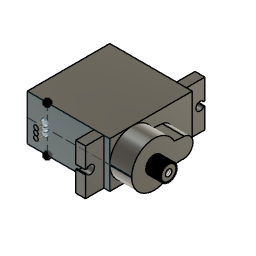
Arm_1 v1 (Autodesk Fusion 360 archive; units mm, degrees)
design "ServoMF90"
Autodesk Fusion 360 part; units mm, degrees
sketch "Sketch1" plane through (0, 0, 0) normal (0, 0, 1) x (1, 0, 0)
  line L0 (-11.3, 11.3) -> (11.3, 11.3)
  line L1 (11.3, 11.3) -> (11.3, -11.3)
  line L2 (11.3, -11.3) -> (-11.3, -11.3)
  line L3 (-11.3, -11.3) -> (-11.3, 11.3)
  line L4 (-11.3, 11.3) -> (11.3, -11.3) construction
  line L5 (11.3, 11.3) -> (-11.3, -11.3) construction
  dimension "d1" = 22.6
  dimension "d2" = 22.6
  constraint horizontal L0
  constraint perpendicular L0 L1
  constraint parallel L0 L2
  constraint parallel L1 L3
  constraint coincident L4 origin
  constraint coincident L5 origin
  measures "d1" distance of L1.end L2.end
  measures "d2" distance of L0.end L1.end
extrude "Extrude1" add sketch "Sketch1" along normal blind 12.5 contours L0 L1 L2 L3 picked at (-3.766667, 3.766667) makes body 1
sketch "Sketch2" plane through (11.3, 0, 0) normal (1, 0, 0) x (0, 1, 0)
  line L0 (-11.3, 0) -> (11.3, 0)
  line L1 (11.3, 0) -> (11.3, 12.5)
  line L2 (11.3, 12.5) -> (-11.3, 12.5)
  line L3 (-11.3, 12.5) -> (-11.3, 0)
  circle A0 centre (-5.148532, 6.347755) radius 6.152245
  line L4 (-5.148532, 6.347755) -> (11.3, 6.25) construction
  circle A1 centre (2.851468, 6.25) radius 2.65
  line L5 (3.075734, 8.890493) -> (0.342379, 9.122646)
  line L6 (3.075734, -8.890493) -> (0.342379, -9.122646)
  line L7 (3.044931, 3.707445) -> (0.309009, 3.507796)
  circle A2 centre (-5.148532, 6.347755) radius 2.3
  dimension "d5" = 5.3
  dimension "d6" = 8
  dimension "d7" = 4.6
  constraint tangent L2 A0
  constraint midpoint L1 L4.end
  constraint tangent A1 L5
  constraint concentric A0 A2
  measures "d5" diameter of A1
  measures "d7" diameter of A2
extrude "Extrude2" add sketch "Sketch2" along normal blind 6 contours A0 A1 | A0 A1 L7 | A0 A1 L5 | A0 A1 | A0 A1 picked at (-0.779294, 7.905006) picked at (0.801754, 3.761707) picked at (0.843844, 8.497494) picked at (0.728856, 6.066378) picked at (2.263353, 5.526518) bodies 1
extrude "Extrude3" add 1 faces at (11.3, -6.264471, 5.742797) along direction (1, 0, 0) blind 10 on bodies 1 bodies 1
sketch "Sketch3" plane through (21.3, 0, 0) normal (1, 0, 0) x (0, 1, 0)
  circle A0 centre (-5.148532, 6.347755) radius 2.3
  circle A1 centre (-5.148532, 6.347755) radius 1.1
  dimension "d12" = 2.2
  constraint concentric A0 A1
  measures "d12" diameter of A1
extrude "Extrude4" cut sketch "Sketch3" against normal blind 4 contours A1 picked at (-5.895648, 6.553327) bodies 1
thread "Thread1" "ISO Metric profile 2.2 M2.2x0.45 6H" major diameter 2.28 minor diameter 1.7754 pitch 0.45 angle 60 resizes the face on face at (19.966667, -4.053998, 6.23823) on bodies 1
sketch "Sketch4" plane through (21.3, 0, 0) normal (1, 0, 0) x (0, 1, 0)
  circle A0 centre (-5.148532, 6.347755) radius 0.8877
  circle A1 centre (-5.148532, 6.347755) radius 2.3
  line L0 (-5.287623, 4.051965) -> (-4.937623, 4.051965)
  line L1 (-4.937623, 4.051965) -> (-4.937623, 4.351965)
  line L2 (-4.937623, 4.351965) -> (-5.287623, 4.351965)
  line L3 (-5.287623, 4.351965) -> (-5.287623, 4.051965)
  line L4 (-4.766335, 4.38397) -> (-4.68869, 4.094192)
  line L5 (-4.428261, 4.474556) -> (-4.766335, 4.38397)
  line L6 (-4.350616, 4.184779) -> (-4.428261, 4.474556)
  line L7 (-4.68869, 4.094192) -> (-4.350616, 4.184779)
  line L8 (-4.271093, 4.549804) -> (-4.121093, 4.289996)
  line L9 (-3.967985, 4.724804) -> (-4.271093, 4.549804)
  line L10 (-3.817985, 4.464996) -> (-3.967985, 4.724804)
  line L11 (-4.121093, 4.289996) -> (-3.817985, 4.464996)
  line L12 (-3.835647, 4.838165) -> (-3.623515, 4.626033)
  line L13 (-3.58816, 5.085653) -> (-3.835647, 4.838165)
  line L14 (-3.376028, 4.873521) -> (-3.58816, 5.085653)
  line L15 (-3.623515, 4.626033) -> (-3.376028, 4.873521)
  line L16 (-3.489672, 5.229403) -> (-3.229865, 5.079403)
  line L17 (-3.314672, 5.532511) -> (-3.489672, 5.229403)
  line L18 (-3.054865, 5.382511) -> (-3.314672, 5.532511)
  line L19 (-3.229865, 5.079403) -> (-3.054865, 5.382511)
  line L20 (-3.256746, 5.696854) -> (-2.966968, 5.619208)
  line L21 (-3.166159, 6.034928) -> (-3.256746, 5.696854)
  line L22 (-2.876381, 5.957282) -> (-3.166159, 6.034928)
  line L23 (-2.966968, 5.619208) -> (-2.876381, 5.957282)
  line L24 (-3.152741, 6.208663) -> (-2.852741, 6.208663)
  line L25 (-3.152741, 6.558663) -> (-3.152741, 6.208663)
  line L26 (-2.852741, 6.558663) -> (-3.152741, 6.558663)
  line L27 (-2.852741, 6.208663) -> (-2.852741, 6.558663)
  line L28 (-3.184746, 6.729951) -> (-2.894969, 6.807597)
  line L29 (-3.275333, 7.068025) -> (-3.184746, 6.729951)
  line L30 (-2.985555, 7.145671) -> (-3.275333, 7.068025)
  line L31 (-2.894969, 6.807597) -> (-2.985555, 7.145671)
  line L32 (-3.35058, 7.225193) -> (-3.090773, 7.375193)
  line L33 (-3.52558, 7.528302) -> (-3.35058, 7.225193)
  line L34 (-3.265773, 7.678302) -> (-3.52558, 7.528302)
  line L35 (-3.090773, 7.375193) -> (-3.265773, 7.678302)
  line L36 (-3.638942, 7.660639) -> (-3.42681, 7.872771)
  line L37 (-3.886429, 7.908126) -> (-3.638942, 7.660639)
  line L38 (-3.674297, 8.120258) -> (-3.886429, 7.908126)
  line L39 (-3.42681, 7.872771) -> (-3.674297, 8.120258)
  line L40 (-4.030179, 8.006614) -> (-3.880179, 8.266422)
  line L41 (-4.333288, 8.181614) -> (-4.030179, 8.006614)
  line L42 (-4.183288, 8.441422) -> (-4.333288, 8.181614)
  line L43 (-3.880179, 8.266422) -> (-4.183288, 8.441422)
  line L44 (-4.497631, 8.239541) -> (-4.419985, 8.529318)
  line L45 (-4.835705, 8.330127) -> (-4.497631, 8.239541)
  line L46 (-4.758059, 8.619905) -> (-4.835705, 8.330127)
  line L47 (-4.419985, 8.529318) -> (-4.758059, 8.619905)
  line L48 (-5.00944, 8.343545) -> (-5.00944, 8.643545)
  line L49 (-5.35944, 8.343545) -> (-5.00944, 8.343545)
  line L50 (-5.35944, 8.643545) -> (-5.35944, 8.343545)
  line L51 (-5.00944, 8.643545) -> (-5.35944, 8.643545)
  line L52 (-5.530728, 8.31154) -> (-5.608373, 8.601318)
  line L53 (-5.868802, 8.220953) -> (-5.530728, 8.31154)
  line L54 (-5.946447, 8.510731) -> (-5.868802, 8.220953)
  line L55 (-5.608373, 8.601318) -> (-5.946447, 8.510731)
  line L56 (-6.02597, 8.145706) -> (-6.17597, 8.405514)
  line L57 (-6.329079, 7.970706) -> (-6.02597, 8.145706)
  line L58 (-6.479079, 8.230514) -> (-6.329079, 7.970706)
  line L59 (-6.17597, 8.405514) -> (-6.479079, 8.230514)
  line L60 (-6.461416, 7.857345) -> (-6.673548, 8.069477)
  line L61 (-6.708903, 7.609857) -> (-6.461416, 7.857345)
  line L62 (-6.921035, 7.821989) -> (-6.708903, 7.609857)
  line L63 (-6.673548, 8.069477) -> (-6.921035, 7.821989)
  line L64 (-6.807391, 7.466107) -> (-7.067198, 7.616107)
  line L65 (-6.982391, 7.162998) -> (-6.807391, 7.466107)
  line L66 (-7.242198, 7.312998) -> (-6.982391, 7.162998)
  line L67 (-7.067198, 7.616107) -> (-7.242198, 7.312998)
  line L68 (-7.040317, 6.998656) -> (-7.330095, 7.076302)
  line L69 (-7.130904, 6.660582) -> (-7.040317, 6.998656)
  line L70 (-7.420682, 6.738228) -> (-7.130904, 6.660582)
  line L71 (-7.330095, 7.076302) -> (-7.420682, 6.738228)
  line L72 (-7.144322, 6.486847) -> (-7.444322, 6.486847)
  line L73 (-7.144322, 6.136847) -> (-7.144322, 6.486847)
  line L74 (-7.444322, 6.136847) -> (-7.144322, 6.136847)
  line L75 (-7.444322, 6.486847) -> (-7.444322, 6.136847)
  line L76 (-7.112317, 5.965559) -> (-7.402094, 5.887913)
  line L77 (-7.02173, 5.627485) -> (-7.112317, 5.965559)
  line L78 (-7.311508, 5.549839) -> (-7.02173, 5.627485)
  line L79 (-7.402094, 5.887913) -> (-7.311508, 5.549839)
  line L80 (-6.946483, 5.470317) -> (-7.20629, 5.320317)
  line L81 (-6.771483, 5.167208) -> (-6.946483, 5.470317)
  line L82 (-7.03129, 5.017208) -> (-6.771483, 5.167208)
  line L83 (-7.20629, 5.320317) -> (-7.03129, 5.017208)
  line L84 (-6.658121, 5.034871) -> (-6.870253, 4.822739)
  line L85 (-6.410634, 4.787383) -> (-6.658121, 5.034871)
  line L86 (-6.622766, 4.575251) -> (-6.410634, 4.787383)
  line L87 (-6.870253, 4.822739) -> (-6.622766, 4.575251)
  line L88 (-6.266884, 4.688896) -> (-6.416884, 4.429088)
  line L89 (-5.963775, 4.513896) -> (-6.266884, 4.688896)
  line L90 (-6.113775, 4.254088) -> (-5.963775, 4.513896)
  line L91 (-6.416884, 4.429088) -> (-6.113775, 4.254088)
  line L92 (-5.799433, 4.455969) -> (-5.877078, 4.166191)
  line L93 (-5.461359, 4.365382) -> (-5.799433, 4.455969)
  line L94 (-5.539004, 4.075605) -> (-5.461359, 4.365382)
  line L95 (-5.877078, 4.166191) -> (-5.539004, 4.075605)
  dimension "d17" = 0.35
  dimension "d18" = 0.3
  dimension "d20" = 360
  constraint horizontal L0
  constraint vertical L1
  constraint horizontal L2
  constraint vertical L3
extrude "Extrude5" cut sketch "Sketch4" against normal blind 4 contours A1 L24 L25 L26 L27 | A1 L20 L21 L22 L23 | A1 L28 L29 L30 L31 | A1 L16 L17 L18 L19 | A1 L32 L33 L34 L35 | A1 L12 L13 L14 L15 | A1 L36 L37 L38 L39 | A1 L8 L9 L10 L11 | A1 L40 L41 L42 L43 | A1 L4 L5 L6 L7 | A1 L44 L45 L46 L47 | A1 L0 L1 L2 L3 | A1 L48 L49 L50 L51 | A1 L92 L93 L94 L95 | A1 L52 L53 L54 L55 | A1 L88 L89 L90 L91 | A1 L56 L57 L58 L59 | A1 L84 L85 L86 L87 | A1 L60 L61 L62 L63 | A1 L80 L81 L82 L83 | A1 L64 L65 L66 L67 | A1 L76 L77 L78 L79 | A1 L68 L69 L70 L71 | A1 L72 L73 L74 L75 picked at (-3.052741, 6.418058) picked at (-3.105958, 5.873232) picked at (-3.142349, 6.958093) picked at (-3.298373, 5.360744) picked at (-3.368675, 7.456534) picked at (-3.616872, 4.915519) picked at (-3.716296, 7.879414) picked at (-4.039752, 4.567899) picked at (-4.16152, 8.197914) picked at (-4.538194, 4.341573) picked at (-4.674008, 8.390329) picked at (-5.078229, 4.251965) picked at (-5.218834, 8.443545) picked at (-5.623055, 4.305181) picked at (-5.758869, 8.353937) picked at (-6.135543, 4.497596) picked at (-6.257311, 8.127611) picked at (-6.580768, 4.816096) picked at (-6.680191, 7.779991) picked at (-6.928388, 5.238976) picked at (-6.998691, 7.334766) picked at (-7.154714, 5.737417) picked at (-7.191105, 6.822278) picked at (-7.244322, 6.277452) bodies 1
sketch "Sketch5" plane through (0, -11.3, 0) normal (0, -1, 0) x (1, 0, 0)
  line L0 (-11.3, 0) -> (11.3, 0)
  line L1 (11.3, 0) -> (11.3, 6.25)
  line L2 (11.3, 6.25) -> (17.3, 6.25)
  line L3 (17.3, 6.25) -> (17.3, 6.44551)
  line L4 (17.3, 6.44551) -> (11.3, 6.44551)
  line L5 (11.3, 6.44551) -> (11.3, 12.5)
  line L6 (11.3, 12.5) -> (-11.3, 12.5)
  line L7 (-11.3, 12.5) -> (-11.3, 0)
  line L8 (17.3, 6.347755) -> (-11.3, 6.25) construction
  line L9 (9.7, 0) -> (7, 0)
  line L10 (7, 0) -> (7, 12.5)
  line L11 (7, 12.5) -> (9.7, 12.5)
  line L12 (9.7, 12.5) -> (9.7, 0)
  dimension "d23" = 2.7
  dimension "d24" = 21
  constraint midpoint L7 L8.end
  constraint horizontal L9
  constraint vertical L10
  constraint horizontal L11
  constraint vertical L12
  constraint coincident L0 L9.start
  measures "d23" distance of L9.start L9.end
  measures "d24" distance of L7 L12
extrude "Extrude6" add sketch "Sketch5" along normal blind 5.05 separate body contours L0 L6 L9 L10 L11 L12 picked at (8.8, 4.166667) makes body 2
sketch "Sketch6" plane through (9.7, 0, 0) normal (1, 0, 0) x (0, 1, 0)
  line L0 (-11.3, 0) -> (-11.3, 12.5)
  line L1 (-11.3, 12.5) -> (-16.35, 12.5)
  line L2 (-16.35, 12.5) -> (-16.35, 0)
  line L3 (-16.35, 0) -> (-11.3, 0)
  line L4 (-16.35, 6.25) -> (-11.3, 6.25) construction
  circle A0 centre (-15.05, 6.25) radius 1.15
  circle A1 centre (-16.35, 6.25) radius 0.6
  dimension "d27" = 2.3
  dimension "d28" = 1.3
  dimension "d30" = 1.2
  constraint midpoint L2 L4.start
  constraint midpoint L0 L4.end
  constraint coincident L4 A0.centre
  constraint coincident L4.start A1.centre
  measures "d27" diameter of A0
  measures "d28" distance of L4.start A0.centre
  measures "d30" diameter of A1
extrude "Extrude7" cut sketch "Sketch6" against normal blind 3 contours L2 A1 | L2 A0 A1 | A0 A1 | A0 A1 picked at (-16.544986, 6.294504) picked at (-16.2991, 6.22375) picked at (-14.520851, 6.306482) picked at (-16.0482, 6.25) bodies 2
mirror "Mirror1" about plane through (0, 0, 0) normal (0, 1, 0) of bodies 2 makes body 3
sketch "Sketch7" plane through (0, -11.3, 0) normal (0, -1, 0) x (1, 0, 0)
  line L0 (-11.3, 0) -> (11.3, 0)
  line L1 (11.3, 0) -> (11.3, 6.25)
  line L2 (11.3, 6.25) -> (17.3, 6.25)
  line L3 (17.3, 6.25) -> (17.3, 6.44551)
  line L4 (17.3, 6.44551) -> (11.3, 6.44551)
  line L5 (11.3, 6.44551) -> (11.3, 12.5)
  line L6 (11.3, 12.5) -> (-11.3, 12.5)
  line L7 (-11.3, 12.5) -> (-11.3, 0)
  line L8 (-11.3, 6.25) -> (17.3, 6.347755) construction
  line L9 (-5.8, 0) -> (-5.8, 12.5) construction
  circle A0 centre (-6.425, 6.25) radius 0.625
  circle A1 centre (-6.424966, 5) radius 0.625
  circle A2 centre (-6.422482, 7.493247) radius 0.625
  dimension "d35" = 5.5
  dimension "d36" = 1.25
  dimension "d38" = 1.25
  dimension "d39" = 1.25
  constraint midpoint L7 L8.start
  constraint coincident L0 L9.start
  constraint coincident L6 L9.end
  constraint perpendicular L6 L9
  measures "d35" distance of L7 L9
  measures "d36" diameter of A0
  measures "d38" diameter of A1
  measures "d39" diameter of A2
extrude "Extrude9" add sketch "Sketch7" along normal blind 2.5 separate body contours A0 A2 | A1 | A0 A2 picked at (-6.46184, 6.041734) picked at (-6.425052, 4.781033) picked at (-6.41129, 7.702519) makes body 4
extrude "Extrude8" [rolled back] along distance 5 taper angle 0
